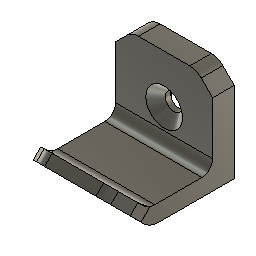
SKADIS_SNS_StandardHook (Autodesk Fusion 360 design; units mm, degrees)
Autodesk Fusion 360 part; units mm, degrees
sketch "HoleTemplate" plane through (0, 0, 0) normal (0, 1, 0) x (1, 0, 0)
  line L0 (20, 25) -> (20, 15) construction
  line L1 (-57.6, 15) -> (-57.6, 25)
  line L2 (-80, 0) -> (0, 0) construction
  arc A0 (77.6, -5) -> (82.4, -5) centre (80, -5) ccw
  arc A1 (97.6, 15) -> (102.4, 15) centre (100, 15) ccw
  arc A2 (-97.6, 25) -> (-102.4, 25) centre (-100, 25) ccw
  line L3 (-82.4, 5) -> (-82.4, -5)
  arc A3 (42.4, 5) -> (37.6, 5) centre (40, 5) ccw
  line L4 (-42.4, 5) -> (-42.4, -5)
  line L5 (60, 25) -> (60, 15) construction
  arc A4 (-77.6, 5) -> (-82.4, 5) centre (-80, 5) ccw
  arc A5 (82.4, 5) -> (77.6, 5) centre (80, 5) ccw
  arc A6 (22.4, 25) -> (17.6, 25) centre (20, 25) ccw
  arc A7 (102.4, 25) -> (97.6, 25) centre (100, 25) ccw
  line L6 (-100, 25) -> (-100, 15) construction
  line L7 (-40, 5) -> (-40, -5) construction
  line L8 (17.6, 15) -> (17.6, 25)
  line L9 (-60, 25) -> (-60, 15) construction
  line L10 (-77.6, -5) -> (-77.6, 5)
  line L11 (102.4, 25) -> (102.4, 15)
  arc A8 (-37.6, 5) -> (-42.4, 5) centre (-40, 5) ccw
  line L12 (-62.4, 25) -> (-62.4, 15)
  line L13 (57.6, 15) -> (57.6, 25)
  line L14 (2.4, -5) -> (2.4, 5)
  line L15 (82.4, 5) -> (82.4, -5)
  line L16 (37.6, -5) -> (37.6, 5)
  arc A9 (62.4, 25) -> (57.6, 25) centre (60, 25) ccw
  line L17 (42.4, 5) -> (42.4, -5)
  arc A10 (-102.4, 15) -> (-97.6, 15) centre (-100, 15) ccw
  line L18 (-37.6, -5) -> (-37.6, 5)
  arc A11 (-82.4, -5) -> (-77.6, -5) centre (-80, -5) ccw
  line L19 (77.6, -5) -> (77.6, 5)
  line L20 (62.4, 25) -> (62.4, 15)
  arc A12 (37.6, -5) -> (42.4, -5) centre (40, -5) ccw
  arc A13 (-22.4, 15) -> (-17.6, 15) centre (-20, 15) ccw
  line L21 (-2.4, 5) -> (-2.4, -5)
  line L22 (-102.4, 25) -> (-102.4, 15)
  line L23 (-22.4, 25) -> (-22.4, 15)
  arc A14 (2.4, 5) -> (-2.4, 5) centre (0, 5) ccw
  line L24 (-97.6, 15) -> (-97.6, 25)
  arc A15 (-17.6, 25) -> (-22.4, 25) centre (-20, 25) ccw
  arc A16 (57.6, 15) -> (62.4, 15) centre (60, 15) ccw
  line L25 (80, 5) -> (80, -5) construction
  arc A17 (-57.6, 25) -> (-62.4, 25) centre (-60, 25) ccw
  line L26 (-17.6, 15) -> (-17.6, 25)
  arc A18 (-62.4, 15) -> (-57.6, 15) centre (-60, 15) ccw
  line L27 (97.6, 15) -> (97.6, 25)
  arc A19 (-2.4, -5) -> (2.4, -5) centre (0, -5) ccw
  arc A20 (17.6, 15) -> (22.4, 15) centre (20, 15) ccw
  arc A21 (-42.4, -5) -> (-37.6, -5) centre (-40, -5) ccw
  line L28 (-80, 5) -> (-80, -5) construction
  line L29 (40, 5) -> (40, -5) construction
  line L30 (0, 5) -> (0, -5) construction
  line L31 (22.4, 25) -> (22.4, 15)
  line L32 (100, 25) -> (100, 15) construction
  line L33 (-20, 25) -> (-20, 15) construction
  line L34 (-2.5, 5) -> (-2.5, -5)
  arc A22 (-2.5, -5) -> (2.5, -5) centre (0, -5) ccw
  line L35 (2.5, -5) -> (2.5, 5)
  arc A23 (2.5, 5) -> (-2.5, 5) centre (0, 5) ccw
  point P0 (-40, 0)
  point P1 (-20, 20)
  dimension "d247" = -40
  dimension "d248" = 0
  dimension "d1" = 10
  dimension "d3" = 2.4
  dimension "d4" = 40
  dimension "d5" = 40
  dimension "d6" = 20
  dimension "d8" = 20
  dimension "d255" = 0.1
  constraint tangent L3 A11
  constraint tangent L10 A11
  constraint parallel L3 L10
  constraint tangent A4 L10
  constraint tangent L3 A4
  constraint vertical L28
  constraint tangent L4 A21
  constraint tangent L18 A21
  constraint parallel L4 L18
  constraint tangent A8 L18
  constraint tangent L4 A8
  constraint vertical L7
  constraint tangent L21 A19
  constraint tangent L14 A19
  constraint parallel L14 L21
  constraint tangent L14 A14
  constraint tangent L21 A14
  constraint parallel L18 L30
  constraint midpoint L2.start L28
  constraint midpoint L2.end L30
  constraint horizontal L2
  constraint equal L7 L30
  constraint equal L7 L28
  constraint midpoint P0 L7
  constraint coincident P0 L2
  constraint equal A8 A14
  constraint equal A4 A8
  constraint coincident L2.end origin
  constraint symmetric L3.start A5.start L30
  constraint symmetric L3.end A0.end L30
  constraint symmetric L10.start A0.start L30
  constraint symmetric A4.start A5.end L30
  constraint symmetric A0 A11 L30
  constraint symmetric A4 A5 L30
  constraint symmetric L4.start A3.start L30
  constraint symmetric L4.end L17.end L30
  constraint symmetric L18.start L16.start L30
  constraint symmetric A8.start A3.end L30
  constraint symmetric A12 A21 L30
  constraint symmetric A3 A8 L30
  constraint tangent A13 L23
  constraint tangent A13 L26
  constraint parallel L23 L26
  constraint tangent A15 L26
  constraint tangent L23 A15
  constraint vertical L33
  constraint equal L30 L33
  constraint equal A14 A15
  constraint midpoint P1 L33
  constraint symmetric A20.end A13.start L30
  constraint symmetric A15.start A6.end L30
  constraint symmetric A6.start L23.start L30
  constraint symmetric L8.start A13.end L30
  constraint symmetric A6 A15 L30
  constraint symmetric A13 A20 L30
  constraint symmetric L13.end L1.end L30
  constraint symmetric L12.start A9.start L30
  constraint symmetric A9 A17 L30
  constraint symmetric L20.end L12.end L30
  constraint symmetric L13.start L1.start L30
  constraint symmetric A16 A18 L30
  constraint symmetric A7.end A2.start L30
  constraint symmetric A7.start A2.end L30
  constraint symmetric A2 A7 L30
  constraint symmetric A1.end A10.start L30
  constraint symmetric A1.start A10.end L30
  constraint symmetric A1 A10 L30
  measures "d1" distance of A14.centre A19.centre
  measures "d3" radius of A14
  measures "d4" distance of L7 L30
  measures "d5" distance of L7 L28
  measures "d6" horizontal distance of A14.centre A13.centre
  measures "d8" vertical distance of L2.end P1
sketch "SH_Profile" plane through (0, 0, 0) normal (1, 0, 0) x (0, 1, 0) in component "SNS_StandardHook_W_D_02"
  line L0 (0, -9) -> (0, 9)
  line L1 (0, 9) -> (-4, 9)
  line L2 (-4, 9) -> (-4, -9)
  line L3 (-4, -9) -> (0, -9)
  line L4 (-4, -9) -> (-15.6284, -9)
  line L5 (-15.6284, -9) -> (-19.4142, -5.2142)
  line L6 (-18, -3.8) -> (-16, -5.8)
  line L7 (-16, -5.8) -> (-4, -5.8)
  line L8 (-4, 0) -> (0, 0) construction
  line L9 (-18, -3.8) -> (-19.4142, -5.2142)
  line L10 (-16, -5.8) -> (-17.4142, -7.2142) construction
  dimension "d14" = 135
  dimension "d16" = 2
  dimension "d17" = 3.2
  dimension "d25" = 4
  dimension "d229" = 12
  dimension "d230" = 2
  dimension "d231" = 9
  dimension "d232" = 18
  constraint vertical L0
  constraint perpendicular L0 L1
  constraint perpendicular L1 L2
  constraint perpendicular L2 L3
  constraint perpendicular L2 L4
  constraint coincident L2 L7.end
  constraint perpendicular L2 L7
  constraint parallel L5 L6
  constraint coincident L2 L8.start
  constraint coincident L0 L8.end
  constraint perpendicular L0 L8
  constraint coincident L5 L9.end
  constraint perpendicular L5 L9
  constraint coincident L5 L10.end
  constraint perpendicular L5 L10
  constraint coincident L8.end origin
  measures "d14" angle of L6 L7
  measures "d16" distance of L5 L6
  measures "d17" distance of L4.end L7
  measures "d25" distance of L0 L2
  measures "d229" distance of L6.end L7.end
  measures "d230" vertical distance of L6.start L6.end
  measures "d231" distance of L1 L8
  measures "d232" distance of L1 L3
extrude "Extrude2" add sketch "SH_Profile" along normal mid plane 18 makes body 1 in component "SNS_StandardHook_W_D_02"
sketch "SH_ScrewHole" plane through (0, 0, 0) normal (0, 1, 0) x (1, 0, 0) in component "SNS_StandardHook_W_D_02"
  circle A0 centre (0, 0) radius 1.6
  circle A1 centre (0, 0) radius 2.6 construction
  line L0 (2.5, -5) -> (2.5, 5)
  arc A2 (2.5, 5) -> (-2.5, 5) centre (0, 5) ccw
  line L1 (-2.5, 5) -> (-2.5, -5)
  arc A3 (-2.5, -5) -> (2.5, -5) centre (0, -5) ccw
  line L2 (0, -6.7) -> (0, 6.7) construction
  line L3 (2.6, -6.7) -> (-2.6, -6.7)
  line L4 (-2.6, -6.7) -> (-2.6, 6.7)
  line L5 (-2.6, 6.7) -> (2.6, 6.7)
  line L6 (2.6, 6.7) -> (2.6, -6.7)
  line L7 (0, -6.7) -> (0, 6.7) construction
  point P0 (0, 5)
  point P1 (0, -5)
  dimension "d31" = 3.2
  dimension "d258" = 5.2
  dimension "d283" = 1.7
  dimension "d284" = 1.7
  dimension "d285" = 5.2
  dimension "d292" = 13.4
  constraint coincident A0.centre A1.centre
  constraint horizontal L3
  constraint vertical L4
  constraint horizontal L5
  constraint vertical L6
  constraint midpoint L3 L2.start
  constraint midpoint L5 L2.end
  constraint midpoint L7 A0.centre
  measures "d31" diameter of A0
  measures "d258" diameter of A1
  measures "d283" distance of L5 P0
  measures "d284" distance of L3 P1
  measures "d285" distance of L3.start L3.end
  measures "d292" distance of L2.end L3
extrude "Extrude3" cut sketch "SH_ScrewHole" against normal up to surface (4 mm away) contours A0 bodies 1 in component "SNS_StandardHook_W_D_02"
extrude "Extrude4" cut sketch "SH_ScrewHole" against normal blind 1.2 contours L0 A2 L1 A3 L3 L5 | L0 A2 A3 L3 L5 L6 | A2 L1 A3 L3 L4 L5 bodies 1 in component "SNS_StandardHook_W_D_02"
chamfer "Chamfer2" distance 3 angle 45 2 edges at (-9, -2, 9) (9, -2, 9) on bodies 1 in component "SNS_StandardHook_W_D_02"
chamfer "Chamfer2" distance 3 angle 45 2 edges at (9, -18.7071, -4.5071) (-9, -18.7071, -4.5071) on bodies 1 in component "SNS_StandardHook_W_D_02"
fillet "Fillet1" radius 4 1 edges at (0, -15.6284, -9) on bodies 1 in component "SNS_StandardHook_W_D_02"
fillet "Fillet1" radius 3 1 edges at (0, -16, -5.8) on bodies 1 in component "SNS_StandardHook_W_D_02"
fillet "Fillet1" radius 2 1 edges at (0, -4, -5.8) on bodies 1 in component "SNS_StandardHook_W_D_02"
fillet "Fillet1" radius 3 4 edges at (-6, -18.7071, -4.5071) (6, -18.7071, -4.5071) (-6, -2, 9) (6, -2, 9) on bodies 1 in component "SNS_StandardHook_W_D_02"
chamfer "Chamfer1" distance 1.8 angle 45 1 edges at (-1.4917, -4, 0.5786) on bodies 1 in component "SNS_StandardHook_W_D_02"
sketch "SH_Profile (2)" plane through (0, 0, 0) normal (1, 0, 0) x (0, 1, 0) in component "SNS_StandardHook_W_D_04"
  line L0 (0, -9) -> (0, 9)
  line L1 (0, 9) -> (-4, 9)
  line L2 (-4, 9) -> (-4, -9)
  line L3 (-4, -9) -> (0, -9)
  line L4 (-4, -9) -> (-15.6284, -9)
  line L5 (-15.6284, -9) -> (-21.4142, -3.2142)
  line L6 (-20, -1.8) -> (-16, -5.8)
  line L7 (-16, -5.8) -> (-4, -5.8)
  line L8 (-4, 0) -> (0, 0) construction
  line L9 (-20, -1.8) -> (-21.4142, -3.2142)
  line L10 (-16, -5.8) -> (-17.4142, -7.2142) construction
  dimension "d14_1" = 135
  dimension "d16_1" = 2
  dimension "d17_1" = 3.2
  dimension "d25_1" = 4
  dimension "d229_1" = 12
  dimension "d230_1" = 4
  dimension "d231_1" = 9
  dimension "d232_1" = 18
  constraint vertical L0
  constraint perpendicular L0 L1
  constraint perpendicular L1 L2
  constraint perpendicular L2 L3
  constraint perpendicular L2 L4
  constraint coincident L2 L7.end
  constraint perpendicular L2 L7
  constraint parallel L5 L6
  constraint coincident L2 L8.start
  constraint coincident L0 L8.end
  constraint perpendicular L0 L8
  constraint coincident L5 L9.end
  constraint perpendicular L5 L9
  constraint coincident L5 L10.end
  constraint perpendicular L5 L10
  constraint coincident L8.end origin
  measures "d14_1" angle of L6 L7
  measures "d16_1" distance of L5 L6
  measures "d17_1" distance of L4.end L7
  measures "d25_1" distance of L0 L2
  measures "d229_1" distance of L6.end L7.end
  measures "d230_1" vertical distance of L6.start L6.end
  measures "d231_1" distance of L1 L8
  measures "d232_1" distance of L1 L3
extrude "Extrude2'" add sketch "SH_Profile (2)" along normal mid plane 18 separate body makes body 2 in component "SNS_StandardHook_W_D_04"
sketch "SH_ScrewHole (2)" plane through (0, 0, 0) normal (0, 1, 0) x (1, 0, 0) in component "SNS_StandardHook_W_D_04"
  circle A0 centre (0, 0) radius 1.6
  circle A1 centre (0, 0) radius 2.6 construction
  line L0 (2.5, -5) -> (2.5, 5)
  arc A2 (2.5, 5) -> (-2.5, 5) centre (0, 5) ccw
  line L1 (-2.5, 5) -> (-2.5, -5)
  arc A3 (-2.5, -5) -> (2.5, -5) centre (0, -5) ccw
  line L2 (0, -6.7) -> (0, 6.7) construction
  line L3 (2.6, -6.7) -> (-2.6, -6.7)
  line L4 (-2.6, -6.7) -> (-2.6, 6.7)
  line L5 (-2.6, 6.7) -> (2.6, 6.7)
  line L6 (2.6, 6.7) -> (2.6, -6.7)
  line L7 (0, -6.7) -> (0, 6.7) construction
  point P0 (0, 5)
  point P1 (0, -5)
  dimension "d31_1" = 3.2
  dimension "d258_1" = 5.2
  dimension "d283_1" = 1.7
  dimension "d284_1" = 1.7
  dimension "d285_1" = 5.2
  dimension "d292_1" = 13.4
  constraint coincident A0.centre A1.centre
  constraint horizontal L3
  constraint vertical L4
  constraint horizontal L5
  constraint vertical L6
  constraint midpoint L3 L2.start
  constraint midpoint L5 L2.end
  constraint midpoint L7 A0.centre
  measures "d31_1" diameter of A0
  measures "d258_1" diameter of A1
  measures "d283_1" distance of L5 P0
  measures "d284_1" distance of L3 P1
  measures "d285_1" distance of L3.start L3.end
  measures "d292_1" distance of L2.end L3
extrude "Extrude3'" cut sketch "SH_ScrewHole (2)" against normal up to surface (4 mm away) contours A0 bodies 2 in component "SNS_StandardHook_W_D_04"
extrude "Extrude4'" cut sketch "SH_ScrewHole (2)" against normal blind 1.2 contours L0 A2 L1 A3 L3 L5 | L0 A2 A3 L3 L5 L6 | A2 L1 A3 L3 L4 L5 bodies 2 in component "SNS_StandardHook_W_D_04"
chamfer "Chamfer2'" distance 3 angle 45 2 edges at (-9, -2, 9) (9, -2, 9) on bodies 2 in component "SNS_StandardHook_W_D_04"
chamfer "Chamfer2'" distance 3 angle 45 2 edges at (9, -20.7071, -2.5071) (-9, -20.7071, -2.5071) on bodies 2 in component "SNS_StandardHook_W_D_04"
fillet "Fillet1'" radius 4 1 edges at (0, -15.6284, -9) on bodies 2 in component "SNS_StandardHook_W_D_04"
fillet "Fillet1'" radius 3 1 edges at (0, -16, -5.8) on bodies 2 in component "SNS_StandardHook_W_D_04"
fillet "Fillet1'" radius 2 1 edges at (0, -4, -5.8) on bodies 2 in component "SNS_StandardHook_W_D_04"
fillet "Fillet1'" radius 3 4 edges at (-6, -20.7071, -2.5071) (6, -20.7071, -2.5071) (-6, -2, 9) (6, -2, 9) on bodies 2 in component "SNS_StandardHook_W_D_04"
chamfer "Chamfer1'" distance 1.8 angle 45 1 edges at (-1.4917, -4, 0.5786) on bodies 2 in component "SNS_StandardHook_W_D_04"
component "SNS_StandardHook_W_D_02" placed x (1, 0, 0) y (0, 1, 0) z (0, 0, 1) at (0, 0, 0)
component "SNS_StandardHook_W_D_04" placed x (1, 0, 0) y (0, 1, 0) z (0, 0, 1) at (0, 0, 0)
equation "Screw_Dia = 3.2 mm"
equation "Layer_Height = 0.2 mm"
equation "Wall_Thickness = 0.4 mm"
equation "d15 = Wall_Thickness * 5"
equation "d16 = d15"
equation "d17 = Wall_Thickness * 8"
equation "HookWidth = 18 mm" comment "default 8mm"
equation "HookDepth = 12 mm"
equation "d29 = HookWidth"
equation "d31 = Screw_Dia"
equation "d229 = HookDepth"
equation "d231 = d232 / 2"
equation "XY_Tolerance = 0.2 mm"
equation "Z_Tolerance = 0.2 mm"
equation "d258 = d31 + 2 mm"
equation "d260 = Layer_Height * 3"
equation "d262 = -Wall_Thickness * 3"
equation "d284 = d283"
equation "d16_1 = d15"
equation "d17_1 = Wall_Thickness * 8"
equation "d29_1 = HookWidth"
equation "d31_1 = Screw_Dia"
equation "d229_1 = HookDepth"
equation "d231_1 = d232_1 / 2"
equation "d258_1 = d31_1 + 2 mm"
equation "d262_1 = -Wall_Thickness * 3"
equation "d284_1 = d283_1"
equation "d159 = ScrewDia"
equation "d165 = PR3D_Wallthickness * 5"
equation "d174 = -PR3D_Wallthickness * 5"
equation "d182 = 3 mm + ( PR3D_Wallthickness * 2.5 )"
equation "d15_1_1 = PR3D_Wallthickness * 5"
equation "d16_1_1 = d15_1_1"
equation "d17_1_1 = PR3D_Wallthickness * 10"
equation "d20_1_1 = SH_HookChamfer"
equation "d22_1_1 = SH_GapWidth"
equation "d29_1_1 = SH_HookWidth"
equation "d31_1_1 = ScrewDia"
equation "d48_1_1 = SH_AdjHookheight"
equation "d49_1 = -PR3D_Wallthickness * 5"
equation "d53_1 = SH_ToolDepth"
equation "d15_2 = PR3D_Wallthickness * 5"
equation "d16_2 = d15_2"
equation "d17_2 = PR3D_Wallthickness * 10"
equation "d20_2 = SH_HookChamfer"
equation "d22_2 = SH_GapWidth"
equation "d29_2 = SH_HookWidth"
equation "d31_2 = ScrewDia"
equation "d48_2 = SH_AdjHookheight"
equation "d15_1_2 = PR3D_Wallthickness * 5"
equation "d16_1_2 = d15_1_2"
equation "d17_1_2 = PR3D_Wallthickness * 8"
equation "d20_1_2 = SH_HookChamfer"
equation "d22_1_2 = SH_GapWidth"
equation "d29_1_2 = SH_HookWidth"
equation "d31_1_2 = ScrewDia"
equation "d48_1_2 = SH_AdjHookheight"
equation "d49_2 = -PR3D_Wallthickness * 5"
equation "d53_2 = SH_ToolDepth"
equation "d197 = PR3D_Wallthickness * 5"
equation "d201 = ( 27 / 2 ) * 1 mm"
equation "d202 = PR3D_Wallthickness * 6"
equation "d204 = PR3D_Wallthickness * 6"
equation "d205 = ( 15 / 2 ) * 1 mm"
equation "d213 = 12 mm"
equation "d215 = ScrewDia"
equation "d216 = d213 / 2"
equation "d221 = -( 18 * 2 ) * 1 mm"
named bodies: "StandardHook_LPR", "StandardHookLPR"
